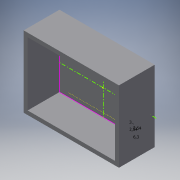
# Autodesk Inventor part: Base Modulo Central
Saved by Autodesk Inventor 2019 (Build 230136000, 136)
## iProperties
Created: 2021-04-15
Part Number: Base Modulo Central
Material: Generic
Document SubType Name: Modeling
Designer: luiza
Density: 1 g/cm^3
Appearance: Default
Author: luiza
Autodesk Inventor part; units mm, degrees
ref_plane "YZ Plane" through (0, 0, 0) normal (1, 0, 0) x (0, 1, 0)
ref_plane "XZ Plane" through (0, 0, 0) normal (0, 1, 0) x (-1, 0, 0)
ref_plane "XY Plane" through (0, 0, 0) normal (0, 0, 1) x (1, 0, 0)
sketch "Sketch1" plane through (0, 0, 0) normal (0, 0, 1) x (1, 0, 0)
  line L0 (-43.815, -27.305) -> (43.815, -27.305) construction
  line L1 (43.815, -27.305) -> (43.815, 27.305) construction
  line L2 (43.815, 27.305) -> (-43.815, 27.305) construction
  line L3 (-43.815, 27.305) -> (-43.815, -27.305) construction
  line L4 (-43.815, -27.305) -> (43.815, 27.305) construction
  line L5 (43.815, -27.305) -> (-43.815, 27.305) construction
  line L6 (-59.8615, -37.305) -> (59.8615, 37.305) construction
  line L7 (59.8615, -37.305) -> (-59.8615, 37.305) construction
  line L8 (-59.8615, -37.305) -> (-59.8615, 52.305)
  line L9 (-59.8615, 52.305) -> (59.8615, 52.305)
  line L10 (59.8615, 52.305) -> (59.8615, -37.305)
  line L11 (-43.815, 27.305) -> (-43.815, 32.305)
  line L12 (59.8615, -37.305) -> (-59.8615, -37.305)
  point P0 (0, 0)
  dimension "d10" = 87.63
  dimension "d11" = 54.61
  dimension "d22" = 5
  dimension "d23" = 20
  constraints: 26 end point, 4 midpoint, 3 parallel, 2 horizontal, 2 perpendicular, 1 point on line, 1 other
  measures "d10" distance of L1.end L2.end
  measures "d11" distance of L0.end L1.end
  measures "d22" distance of L2.end L11.end
  measures "d23" distance from line of L9 L11.end
extrude "Extrusion1" add sketch "Sketch1" against normal blind 5
sketch "Sketch2" plane through (0, 0, 0) normal (0, 0, 1) x (1, 0, 0)
  line L0 (59.8615, -37.305) -> (59.8615, 52.305) projected
  line L1 (59.8615, 52.305) -> (-59.8615, 52.305) projected
  line L2 (-59.8615, 52.305) -> (-59.8615, -37.305) projected
  line L3 (-59.8615, -37.305) -> (59.8615, -37.305) projected
  line L4 (54.8615, 47.305) -> (54.8615, -32.305)
  line L5 (54.8615, -32.305) -> (-54.8615, -32.305)
  line L6 (-54.8615, -32.305) -> (-54.8615, 47.305)
  line L7 (-54.8615, 47.305) -> (54.8615, 47.305)
  dimension "d24" = 5
  constraints: 8 end point, 3 other
  measures "d24" distance between parallel lines of L0 L4
extrude "Extrusion2" add sketch "Sketch2" along normal blind 40
sketch "Sketch3" plane through (0, 0, 0) normal (0, 0, 1) x (1, 0, 0)
  line L0 (-54.8615, 32.305) -> (-54.8615, -32.305) projected
  line L1 (-54.8615, -32.305) -> (54.8615, -32.305) projected
  line L2 (54.8615, -32.305) -> (54.8615, 32.305) projected
  line L3 (54.8615, 32.305) -> (-54.8615, 32.305) projected
  circle A0 centre (41.275, -24.765) radius 1.5
  line L4 (-43.815, -27.305) -> (43.815, -27.305) construction
  line L5 (43.815, -27.305) -> (43.815, 27.305) construction
  line L6 (0, -39.0866) -> (0, 42.4673)
  line L7 (66.4004, 0) -> (-64.4069, 0)
  circle A1 centre (41.275, -24.765) radius 6.3 construction
  line L8 (44.425, -30.221) -> (38.125, -30.221)
  line L9 (38.125, -30.221) -> (34.975, -24.765)
  line L10 (34.975, -24.765) -> (38.125, -19.309)
  line L11 (38.125, -19.309) -> (44.425, -19.309)
  line L12 (44.425, -19.309) -> (47.575, -24.765)
  line L13 (44.425, -30.221) -> (47.575, -24.765)
  line L14 (31.8377, -24.765) -> (36.5564, -32.9379)
  line L15 (36.5564, -32.9379) -> (45.9936, -32.9379)
  line L16 (45.9936, -32.9379) -> (50.7123, -24.765)
  line L17 (50.7123, -24.765) -> (45.9936, -16.5921)
  line L18 (45.9936, -16.5921) -> (36.5564, -16.5921)
  line L19 (36.5564, -16.5921) -> (31.8377, -24.765)
  point P0 (0, 0)
  dimension "d17" = 2.54
  dimension "d18" = 2.54
  dimension "d19" = 3
  dimension "d20" = 6.3
  constraints: 28 end point, 6 point on circle, 4 parallel, 3 equal length, 2 centre point, 2 horizontal, 1 coincident, 1 vertical, 5 other
  measures "d17" distance from line of L4 A0.centre
  measures "d18" distance from line of L5 A0.centre
  measures "d19" diameter of A0
  measures "d20" distance of L8.start L8.end
body "Solid1"
